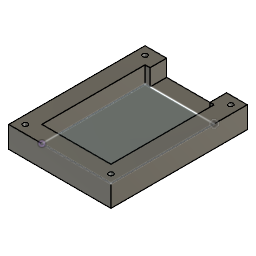
Hackpad bottom piece (Autodesk Fusion 360 design; units mm, degrees)
part number: 2026-02-04-17-29-22-272
Autodesk Fusion 360 part; units mm, degrees
sketch "Sketch1" plane through (0, 0, 0) normal (0, 0, 1) x (1, 0, 0)
  line L0 (0, 0) -> (41.5, 0)
  line L1 (41.5, 0) -> (41.5, 62)
  line L2 (41.5, 62) -> (0, 62)
  line L3 (0, 62) -> (0, 0)
  line L4 (-10, -10) -> (51.5, -10)
  line L5 (51.5, -10) -> (51.5, 72)
  line L6 (51.5, 72) -> (-10, 72)
  line L7 (-10, 72) -> (-10, -10)
  circle A0 centre (-5, 67) radius 1.45
  circle A1 centre (46.5, 67) radius 1.45
  circle A2 centre (46.5, -5) radius 1.45
  circle A3 centre (-5, -5) radius 1.45
  dimension "d1" = 41.5
  dimension "d2" = 62
  dimension "d3" = 10
  dimension "d4" = 10
  dimension "d5" = 10
  dimension "d6" = 10
  dimension "d7" = 2.9
  dimension "d8" = 5
  dimension "d9" = 5
  dimension "d10" = 2.9
  dimension "d11" = 5
  dimension "d12" = 5
  dimension "d13" = 2.9
  dimension "d14" = 5
  dimension "d15" = 5
  dimension "d16" = 2.9
  dimension "d17" = 5
  dimension "d18" = 5
  constraint horizontal L0
  constraint vertical L1
  constraint horizontal L2
  constraint vertical L3
  constraint coincident L0.start L3.end
  constraint horizontal L4
  constraint vertical L5
  constraint horizontal L6
  constraint vertical L7
  measures "d1" distance of L0.start L0.end
  measures "d2" distance of L0.start L2.end
  measures "d3" distance of L1 L5
  measures "d4" distance of L3 L7
  measures "d5" distance of L0 L4
  measures "d6" distance of L2 L6
  measures "d7" diameter of A0
  measures "d8" distance of L6 A0.centre
  measures "d9" distance of L7 A0.centre
  measures "d10" diameter of A1
  measures "d11" distance of L6 A1.centre
  measures "d12" distance of L5 A1.centre
  measures "d13" diameter of A2
  measures "d14" distance of L5 A2.centre
  measures "d15" distance of L4 A2.centre
  measures "d16" diameter of A3
  measures "d17" distance of L7 A3.centre
  measures "d18" distance of L4 A3.centre
extrude "Extrude2" add sketch "Sketch1" along normal blind 3 contours L0 L1 L2 L3
extrude "Extrude3" add sketch "Sketch1" along normal blind 13
sketch "PCB Example" plane through (0, 0, 3) normal (0, 0, 1) x (-1, 0, 0)
  line L0 (0, -62) -> (0, 0)
  line L1 (0, 0) -> (-41.5, 0)
  line L2 (-41.5, 0) -> (-41.5, -62)
  line L3 (-41.5, -62) -> (0, -62)
  line L4 (0, 0) -> (-41.5, 0)
  line L5 (-41.5, 0) -> (-41.5, -62)
  line L6 (-41.5, -62) -> (0, -62)
  line L7 (0, -62) -> (0, 0)
  constraint horizontal L4
  constraint vertical L5
  constraint horizontal L6
  constraint vertical L7
  constraint coincident L2.end L3.start
  constraint coincident L0.end L1.start
sketch "Sketch5" plane through (0, 0, 0) normal (0, 0, 1) x (1, 0, 0)
  line L0 (2, 4) -> (21, 4) construction
  line L1 (21, 4) -> (21, 0) construction
  line L2 (21, 0) -> (2, 0) construction
  line L3 (2, 0) -> (2, 4) construction
  dimension "d27" = 2
  text T0 "Idelles Hackpad" font "Arial" height 2 align left top in box 19 x 4 at (2, 4) x (1, 0) y (0, -1) spacing 1
extrude "Extrude4" add sketch "Sketch5" against normal blind 1 text T0
sketch "Sketch6" plane through (0, 0, 0) normal (0, 0, 1) x (1, 0, 0)
  line L0 (3, 62) -> (39, 62)
  line L1 (39, 62) -> (39, 72)
  line L2 (39, 72) -> (3, 72)
  line L3 (3, 72) -> (3, 62)
  constraint horizontal L0
  constraint vertical L1
  constraint horizontal L2
  constraint vertical L3
extrude "Extrude5" cut sketch "Sketch6" along normal blind 13
sketch "Sketch7" plane through (0, 0, 0) normal (0, 0, 1) x (1, 0, 0)
  line L0 (3, 62) -> (39, 62)
  line L1 (39, 62) -> (39, 72)
  line L2 (39, 72) -> (3, 72)
  line L3 (3, 72) -> (3, 62)
  constraint horizontal L0
  constraint vertical L1
  constraint horizontal L2
  constraint vertical L3
extrude "Extrude6" add sketch "Sketch7" along normal blind 3
sketch "Sketch8" plane through (0, 0, 0) normal (0, 0, 1) x (1, 0, 0)
sketch "Sketch9" plane through (0, 0, 0) normal (0, 0, 1) x (1, 0, 0)
sketch "Sketch10" plane through (0, 0, 0) normal (0, 0, 1) x (1, 0, 0)
sketch "Sketch11" plane through (0, 0, 0) normal (0, 1, 0) x (1, 0, 0)
sketch "Sketch12" plane through (0, 0, 0) normal (0, 0, 1) x (1, 0, 0)
sketch "Sketch13" plane through (0, 0, 0) normal (0, 0, 1) x (1, 0, 0)
equation "d28 = 'Idelles Hackpad'"
